TopBearing_v2 (Autodesk Fusion 360 design; units mm, degrees)
Autodesk Fusion 360 part; units mm, degrees
sketch "Sketch1" plane through (0, 0, 0) normal (0, 0, 1) x (1, 0, 0)
  circle A0 centre (0, 0) radius 34.5
  circle A1 centre (0, 0) radius 13
  dimension "OuterLip" = 69
  dimension "InnerLip" = 26
  constraint coincident A0.centre A1.centre
  constraint concentric A0 A1
  measures "OuterLip" diameter of A0
  measures "InnerLip" diameter of A1
extrude "Extrude1" add sketch "Sketch1" along normal blind 8
sketch "Sketch2" plane through (0, 0, 8) normal (0, 0, 1) x (-1, 0, 0)
  circle A0 centre (0, 0) radius 13
  circle A1 centre (0, 0) radius 34.5
  circle A2 centre (0, 0) radius 32.5
  circle A3 centre (0, 0) radius 16
  dimension "OuterBearingDia" = 65
  dimension "InnerBearingDia" = 32
  constraint coincident A0.centre A1.centre
  constraint concentric A2 A3
  measures "OuterBearingDia" diameter of A2
  measures "InnerBearingDia" diameter of A3
extrude "Extrude2" cut sketch "Sketch2" against normal blind 6
sketch "Sketch3" plane through (0, 0, 8) normal (0, 0, 1) x (-1, 0, 0)
  circle A0 centre (0, 0) radius 32.5
  circle A1 centre (0, 0) radius 16
  circle A2 centre (0, 0) radius 28 construction
  circle A3 centre (0, -28) radius 2
  circle A4 centre (0, -28) radius 4.24
  dimension "d10" = 56
  dimension "d13" = 4
  dimension "d15" = 8.48
  constraint coincident A0.centre A1.centre
  constraint coincident A2 A3.centre
  constraint concentric A3 A4
  measures "d10" diameter of A2
  measures "d13" diameter of A3
  measures "d15" diameter of A4
extrude "Extrude3" cut sketch "Sketch3" against normal through all contours A3
extrude "Extrude4" add sketch "Sketch3" along normal blind 5 contours A4
chamfer "Chamfer1" distance 4 angle 45 1 edges at (3.9531, 26.4668, 8)
pattern_circular "C-Pattern1" count 5 over 360 about axis through (0, 0, 11) along (0, 0, -1) of "Extrude3", "Extrude4", "Chamfer1"
equation "BoltHoleDia = ( 28 * 2 ) * 1 mm"
equation "d10 = BoltHoleDia"
equation "M4BoltHole = 4 mm"
equation "BoltWall = 8.48 mm"
equation "d13 = M4BoltHole"
equation "d15 = BoltWall"
